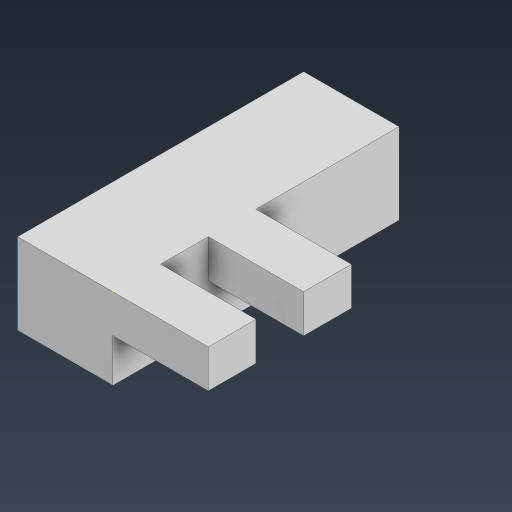
# Autodesk Inventor part: millenium
Saved by Autodesk Inventor 2024 (Build 280153000, 153)
## iProperties
Created: 2023-12-26
Part Number: millenium
Material: Generic
Document SubType Name: Modeling
Designer: Piter
Density: 1 g/cm^3
Appearance: Default
Author: Piter
Autodesk Inventor part; units mm, degrees
ref_plane "YZ Plane" through (0, 0, 0) normal (1, 0, 0) x (0, 1, 0)
ref_plane "XZ Plane" through (0, 0, 0) normal (0, 1, 0) x (-1, 0, 0)
ref_plane "XY Plane" through (0, 0, 0) normal (0, 0, 1) x (1, 0, 0)
sketch "Sketch1" plane through (0, 0, 0) normal (0, 1, 0) x (-1, 0, 0)
  line L0 (0, 0) -> (20, 0)
  line L1 (20, 0) -> (20, -60)
  line L2 (20, -60) -> (0, -60)
  line L3 (0, -60) -> (0, 0)
  dimension "d0" = 20
  dimension "d1" = 60
  constraints: 8 end point, 2 parallel, 1 horizontal, 1 perpendicular
  measures "d0" distance of L1.end L2.end
  measures "d1" distance of L0.end L1.end
extrude "Extrusion1" add sketch "Sketch1" along normal blind 17
sketch "Sketch2" plane through (0, 0, 0) normal (1, 0, 0) x (0, 0, -1)
  line L0 (60, 17) -> (0, 17) projected
  line L1 (0, 17) -> (10, 17)
  line L2 (10, 17) -> (10, 9)
  line L3 (10, 9) -> (0, 9)
  line L4 (0, 9) -> (0, 17)
  line L5 (10, 17) -> (20, 17)
  line L6 (20, 17) -> (30, 17)
  line L7 (30, 17) -> (30, 9)
  line L8 (30, 9) -> (20, 9)
  line L9 (20, 9) -> (20, 17)
  point P0 (0, 0)
  dimension "d4" = 10
  dimension "d5" = 8
  dimension "d6" = 10
  dimension "d7" = 10
  dimension "d8" = 8
  constraints: 18 end point, 4 parallel, 2 horizontal, 2 perpendicular, 1 point on line
  measures "d4" distance of L2.end L3.end
  measures "d5" distance of L1.end L2.end
  measures "d6" distance of L1.end L5.end
  measures "d7" distance of L7.end L8.end
  measures "d8" distance of L6.end L7.end
extrude "Extrusion2" add sketch "Sketch2" along normal blind 20
sketch "Sketch3" plane through (0, 17, 0) normal (0, 1, 0) x (1, 0, 0)
  point P0 (0, 0)
body "Solid1"
